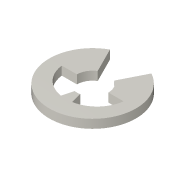
# Autodesk Inventor part: clamp_ring
Saved by Autodesk Inventor 2016 SP1 (Build 200210100, 210)
## iProperties
Created: 2018-07-05
Part Number: clamp_ring
Material: Stahl, geschmiedet
Document SubType Name: Modeling
Designer: WhoTheHeck
Density: 7.85 g/cm^3
Appearance: Stahl
Author: WhoTheHeck
Autodesk Inventor part; units mm, degrees
ref_plane "YZ Plane" through (0, 0, 0) normal (1, 0, 0) x (0, 1, 0)
ref_plane "XZ Plane" through (0, 0, 0) normal (0, 1, 0) x (-1, 0, 0)
ref_plane "XY Plane" through (0, 0, 0) normal (0, 0, 1) x (1, 0, 0)
sketch "Skizze1" plane through (0, 0, 0) normal (0, 0, 1) x (1, 0, 0)
  circle A0 centre (0, 0) radius 2
  dimension "d0" = 4
  constraints: 1 centre point, 1 coincident
  measures "d0" diameter of A0
extrude "Extrusion1" add sketch "Skizze1" along normal blind 0.4
sketch "Skizze2" plane through (0, 0, 0.4) normal (0, 0, 1) x (1, 0, 0)
  circle A0 centre (0, 0) radius 0.725
  line L0 (-0.3824, 0.616) -> (-0.9563, 1.7566)
  circle A1 centre (0, 0) radius 2 projected
  line L1 (0.3824, 0.616) -> (0.9563, 1.7566)
  line L2 (-0.725, 0) -> (-1.425, 0)
  line L3 (-0.1097, -0.7167) -> (-0.2437, -1.2167)
  arc A2 (-1.425, 0) -> (-0.2437, -1.2167) centre (-0.0351, 0.1677) ccw
  line L4 (0.725, 0) -> (1.425, 0)
  line L5 (0.1386, -0.7116) -> (0.2726, -1.2116)
  arc A3 (0.2726, -1.2116) -> (1.425, 0) centre (0.0351, 0.1681) ccw
  line L6 (0, 0) -> (2, 0) construction
  line L7 (0, 0) -> (-2, 0) construction
  dimension "d3" = 1.45
  dimension "d4" = 1.4
  dimension "d5" = 1.4
  dimension "d6" = 75
  dimension "d7" = 75
  dimension "d8" = 0.7
  dimension "d9" = 0.7
  dimension "d10" = 0.5
  dimension "d11" = 0.5
  constraints: 16 end point, 14 point on circle, 3 centre point, 3 horizontal, 2 collinear, 1 coincident, 1 point on line
  measures "d3" diameter of A0
  measures "d4" radius of A3
  measures "d5" radius of A2
  measures "d6" angle of L7 L3
  measures "d7" angle of L6 L5
  measures "d8" distance of L4.start L4.end
  measures "d9" distance of L2.start L2.end
  measures "d10" vertical distance of L3.start L3.end
  measures "d11" vertical distance of L5.start L5.end
extrude "Extrusion2" cut sketch "Skizze2" against normal through all contours A0 | L4 A3 L5 A0 | A0 L0 A1 L1 | L3 A2 L2 A0
equation "\"d5\" = d4"
equation "\"d7\" = d6"
equation "\"d9\" = d8"
equation "\"d11\" = d10"
